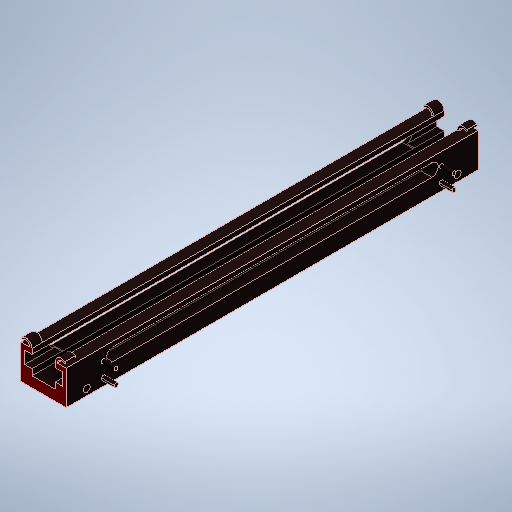
# Autodesk Inventor part: Rack ( Female Fixation )
Saved by Autodesk Inventor 2025.4 (Build 294407000, 407)
## iProperties
Created: 2026-03-18
Part Number: Rack ( Female Fixation )
Material: Generic
Document SubType Name: Modeling
Designer: lenovo
Density: 1 g/cm^3
Appearance: Default(2)
Author: lenovo
Autodesk Inventor part; units mm, degrees
ref_plane "YZ Plane" through (0, 0, 0) normal (1, 0, 0) x (0, 1, 0)
ref_plane "XZ Plane" through (0, 0, 0) normal (0, 1, 0) x (-1, 0, 0)
ref_plane "XY Plane" through (0, 0, 0) normal (0, 0, 1) x (1, 0, 0)
sketch "Sketch1" plane through (0, 0, 0) normal (0, 0, 1) x (1, 0, 0)
  line L0 (-11, -8.3) -> (11, -8.3)
  line L1 (11, -8.3) -> (11, 8.3)
  line L2 (11, 8.3) -> (-11, 8.3)
  line L3 (-11, 8.3) -> (-11, -8.3)
  line L4 (-11, -8.3) -> (11, 8.3) construction
  line L5 (11, -8.3) -> (-11, 8.3) construction
  line L6 (-5.6, 8.3) -> (-5.6, 5.8)
  line L7 (-5.6, 5.8) -> (-9.1, 5.8)
  line L8 (-9.1, 5.8) -> (-9.1, -0.2)
  line L9 (-9.1, -0.2) -> (-5.6, -0.2)
  line L10 (-5.6, -0.2) -> (-5.6, -3.2)
  line L11 (-5.6, -3.2) -> (0, -3.2)
  line L12 (0, 8.3) -> (0, -8.3) construction
  line L13 (5.6, 8.3) -> (5.6, 5.8)
  line L14 (5.6, 5.8) -> (9.1, 5.8)
  line L15 (9.1, 5.8) -> (9.1, -0.2)
  line L16 (9.1, -0.2) -> (5.6, -0.2)
  line L17 (5.6, -0.2) -> (5.6, -3.2)
  line L18 (5.6, -3.2) -> (0, -3.2)
  point P0 (0, 0)
  point P1 (-5.6, 7.05)
  point P2 (-5.6, -1.7)
  point P3 (5.6, 8.3)
  dimension "d0" = 22
  dimension "d1" = 16.6
  dimension "d3" = 5.6
  dimension "d4" = 2.5
  dimension "d5" = 6
  dimension "d6" = 3
  dimension "d7" = 3.5
  dimension "d36" = 18.2
  constraints: 38 end point, 7 perpendicular, 6 midpoint, 6 symmetric about line, 2 parallel, 2 point on line, 1 horizontal, 1 vertical alignment
  measures "d0" distance of L1.end L2.end
  measures "d1" distance between parallel lines of L0 L2
  measures "d3" distance between parallel lines of L6 L12
  measures "d4" distance of L6.start L6.end
  measures "d5" distance of L7.end L8.end
  measures "d6" distance of L9.end L10.end
  measures "d7" distance between parallel lines of L6 L8
  measures "d36" distance between parallel lines of L15 L8
extrude "Extrusion1" add sketch "Sketch1" along normal mid plane 200 contours L3 L2 L6 L7 L8 L9 L10 L11 L18 L17 L16 L15 L14 L13 L1 L0
sketch "Sketch2" plane through (11, -8.3, 100) normal (1, 0, 0) x (0, 0, -1)
  line L0 (200, 16.6) -> (200, 0) projected
  line L1 (200, 0) -> (0, 0) projected
  circle A0 centre (190, 3) radius 1.65
  line L2 (0, 0) -> (0, 16.6) projected
  line L3 (200, 16.6) -> (0, 16.6) projected
  line L4 (100, 16.6) -> (100, 0)
  circle A1 centre (10, 3) radius 1.65
  point P0 (100, 8.3)
  dimension "d13" = 3.3
  dimension "d18" = 180
  dimension "d19" = 3
  constraints: 2 centre point, 2 end point, 2 midpoint, 1 symmetric about line, 1 other
  measures "d13" diameter of A0
  measures "d18" diameter of A0.centre L4
  measures "d19" distance from line of L1 A0.centre
extrude "Extrusion2" cut sketch "Sketch2" against normal blind 180 contours A0 | A1
sketch "Sketch5" plane through (-11, -8.3, 100) normal (-1, 0, 0) x (0, 0, 1)
  line L0 (-185, 11.1) -> (-15, 11.1) construction
  line L1 (-185, 8.05) -> (-15, 8.05)
  line L2 (-15, 14.15) -> (-185, 14.15)
  arc A0 (-185, 14.15) -> (-185, 8.05) centre (-185, 11.1) ccw
  arc A1 (-15, 8.05) -> (-15, 14.15) centre (-15, 11.1) ccw
  line L3 (-200, 14.1) -> (-200, 8.1) projected
  line L4 (-200, 0) -> (0, 0) projected
  line L5 (-200, 16.6) -> (0, 16.6) projected
  line L6 (-100, 16.6) -> (-100, 8.05)
  point P0 (-100, 8.3)
  point P1 (-100, 11.1)
  point P2 (-200, 11.1)
  point P3 (-100, 0)
  dimension "d23" = 85
  dimension "d24" = 6.1
  constraints: 10 end point, 5 midpoint, 4 point on circle, 4 tangent, 2 centre point, 1 horizontal, 1 horizontal alignment, 1 parallel, 1 vertical alignment
  measures "d23" distance of point (-100, 11.1) L0.end
  measures "d24" diameter of A1
extrude "Extrusion4" cut sketch "Sketch5" against normal up to next
sketch "Sketch6" plane through (0, 0, 100) normal (0, 0, 1) x (1, 0, 0)
  line L0 (-11, 8.3) -> (-5.6, 8.3) projected
  arc A0 (-6.6, 8.3) -> (-9.8, 9.9) centre (-8.6, 8.3) ccw
  line L1 (-5.6, 8.3) -> (-11, 8.3) projected
  arc A1 (-5.6, 8.3) -> (-10.4, 10.7) centre (-8.6, 8.3) ccw
  arc A2 (-10.4, 10.7) -> (-9.8, 9.9) centre (-10.1, 10.3) ccw
  line L2 (-11, 8.3) -> (-11, -8.3) projected
  point P0 (0, 0)
  point P1 (-6.5, 8.3)
  dimension "d29" = 2
  dimension "d31" = 1
  dimension "d32" = 2
  constraints: 6 point on circle, 3 centre point, 3 point on line, 2 tangent
  measures "d29" radius of A0
  measures "d31" radial gap between concentric circles of A0 A1
  measures "d32" distance from line of L0 A2.centre
extrude "Extrusion5" add sketch "Sketch6" against normal blind 5
mirror "Mirror1" about plane through (0, 0, 0) normal (1, 0, 0) of "Extrusion5"
mirror "Mirror2" about plane through (0, 0, 0) normal (0, 0, 1) of "Extrusion5", "Mirror1"
mirror "Mirror3" about plane through (0, 0, 0) normal (1, 0, 0) of "Extrusion4"
sketch "Sketch7" plane through (11, -8.3, 100) normal (1, 0, 0) x (0, 0, -1)
  line L0 (170, 11.1) -> (185, 11.1) construction
  line L1 (170, 8.05) -> (185, 8.05)
  line L2 (185, 14.15) -> (170, 14.15)
  arc A0 (170, 14.15) -> (170, 8.05) centre (170, 11.1) ccw
  arc A1 (185, 8.05) -> (185, 14.15) centre (185, 11.1) ccw
  arc A2 (185, 8.05) -> (185, 14.15) centre (185, 11.1) ccw projected
  arc A3 (177.5, 8.05) -> (177.5, 14.15) centre (177.5, 11.1) ccw
  point P0 (100, 8.3)
  dimension "d37" = 15
  constraints: 8 end point, 6 point on circle, 4 tangent, 3 centre point, 3 midpoint, 2 concentric, 2 vertical alignment, 1 coincident, 1 horizontal, 1 parallel
  measures "d37" distance of L0.end L0.start
extrude "Extrusion6" add sketch "Sketch7" against normal up to surface (5.4 mm away) contours A3 L2 A1 L1
sketch "Sketch8" plane through (11, -8.3, 100) normal (1, 0, 0) x (0, 0, -1)
  circle A0 centre (182, 10.6) radius 0.95
  circle A1 centre (182, 3.6) radius 1.05
  line L0 (181.05, 4.0472) -> (181.05, 3.1528)
  line L1 (182, 4.65) -> (182, 2.55)
  line L2 (182.95, 4.0472) -> (182.95, 3.1528)
  line L3 (0, 16.6) -> (200, 16.6) projected
  line L4 (200, 16.6) -> (200, 0) projected
  point P0 (100, 8.3)
  point P1 (182.95, 3.1528)
  point P2 (182.95, 4.0472)
  dimension "d40" = 1.9
  dimension "d41" = 2.1
  dimension "d42" = 1.9
  dimension "d43" = 7
  dimension "d44" = 6
  dimension "d45" = 18
  constraints: 6 end point, 4 point on circle, 2 centre point, 2 symmetric about line, 1 coincident, 1 midpoint, 1 vertical, 1 vertical alignment
  measures "d40" diameter of A0
  measures "d41" diameter of A1
  measures "d42" distance between parallel lines of L0 L2
  measures "d43" distance of A1.centre A0.centre
  measures "d44" distance from line of L3 A0.centre
  measures "d45" distance from line of L4 A1.centre
extrude "Extrusion7" add sketch "Sketch8" along normal blind 6.2 contours A0 | L2 A1 L1 | L1 A1 L0
mirror "Mirror4" about plane through (0, 0, 0) normal (0, 0, 1) of "Extrusion6", "Extrusion7"
ref_plane "Work Plane1" through (0, 0, 0) normal (1, 0, 0) x (0, 1, 0)
ref_plane "Work Plane2" through (0, 0, 0) normal (-1, 0, 0) x (0, 1, 0)
ref_plane "Work Plane3" through (0, 0, 0) normal (-1, 0, 0) x (0, 1, 0)
equation "\"d15\" = d18"
body "Solid1"
